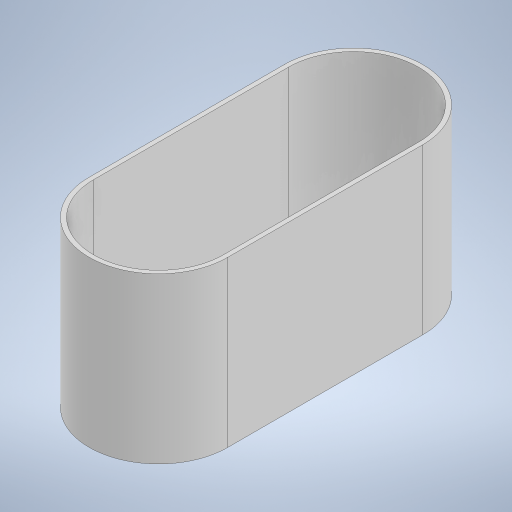
# Autodesk Inventor part: Cinta
Saved by Autodesk Inventor 2023 (Build 270158000, 158)
## iProperties
Created: 2023-04-20
Part Number: Cinta
Material: Genérico
Document SubType Name: Modeling
Designer: sergi
Density: 1 g/cm^3
Appearance: Valor por defecto
Author: sergi
Autodesk Inventor part; units mm, degrees
ref_plane "YZ Plane" through (0, 0, 0) normal (1, 0, 0) x (0, 1, 0)
ref_plane "XZ Plane" through (0, 0, 0) normal (0, 1, 0) x (-1, 0, 0)
ref_plane "XY Plane" through (0, 0, 0) normal (0, 0, 1) x (1, 0, 0)
sketch "Boceto1" plane through (0, 0, 0) normal (0, 1, 0) x (-1, 0, 0)
  arc A0 (16, 0) -> (-16, 0) centre (0, 0) ccw
  line L0 (0, 0) -> (45, 0) construction
  arc A1 (-16, -45) -> (16, -45) centre (0, -45) ccw
  line L1 (16, 0) -> (16, -45)
  line L2 (-16, -45) -> (-16, 0)
  arc A2 (15, 0) -> (-15, 0) centre (0, 0) ccw
  arc A3 (-15, -45) -> (15, -45) centre (0, -45) ccw
  line L3 (15, 0) -> (15, -45)
  line L4 (-15, -45) -> (-15, 0)
  dimension "d0" = 32
  dimension "d3" = 32
  dimension "d4" = 30
  dimension "d5" = 30
  constraints: 10 end point, 8 point on circle, 4 centre point, 4 tangent, 3 coincident, 2 perpendicular, 2 point on line, 1 horizontal, 1 parallel
  measures "d0" diameter of A0
  measures "d3" diameter of A1
  measures "d4" diameter of A2
  measures "d5" diameter of A3
extrude "Extrusión1" add sketch "Boceto1" along normal blind 38
